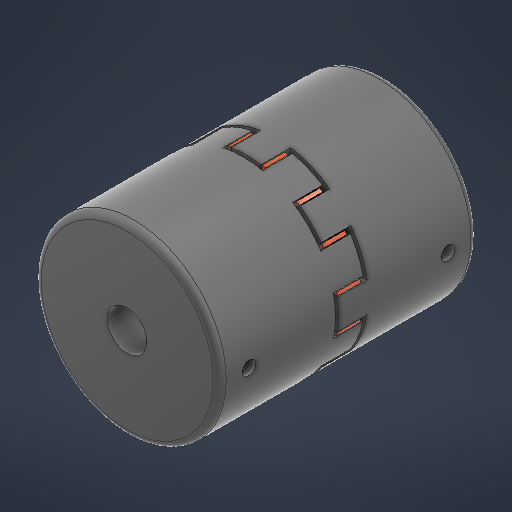
# Autodesk Inventor part: Accouplement12-25
Saved by Autodesk Inventor 2026.2 (Build 302298010, 298A)
## iProperties
Created: 2026-04-18
Part Number: Accouplement12-25
Material: Générique
Document SubType Name: Modeling
Designer: romai
Density: 1 g/cm^3
Appearance: Par défaut
Author: romai
Autodesk Inventor part; units mm, degrees
note: some values were not read from the file. Chosen so that the rebuilt part matches the saved one: direction of "Perçage5".
sketch "Esquisse1" plane through (0, 0, 0) normal (0, 0, 1) x (1, 0, 0)
  circle A0 centre (0, 0) radius 28
  dimension "d0" = 56
  constraints: 1 centre point, 1 coincident
  measures "d0" diameter of A0
extrude "Extrusion1" add sketch "Esquisse1" against normal blind 44
sketch "Esquisse2" plane through (0, 0, 0) normal (0, 0, 1) x (1, 0, 0)
  point P0 (0, 0)
  point P1 (0, 0)
  constraints: 1 coincident
hole "Perçage1" at (0, 0, 0) direction (0, 0, -1) diameter 12 depth 22
sketch "Esquisse4" plane through (0, 0, -44) normal (0, 0, -1) x (-1, 0, 0)
  line L0 (-6, 40) -> (6, 40)
  line L1 (6, 40) -> (6, -40)
  line L2 (6, -40) -> (-6, -40)
  line L3 (-6, -40) -> (-6, 40)
  line L4 (-6, 40) -> (6, -40) construction
  line L5 (6, 40) -> (-6, -40) construction
  line L6 (-32.5269, 24.0416) -> (-24.0416, 32.5269)
  line L7 (24.0416, -32.5269) -> (-32.5269, 24.0416)
  line L8 (-24.0416, 32.5269) -> (32.5269, -24.0416)
  line L9 (32.5269, -24.0416) -> (24.0416, -32.5269)
  line L10 (-40, -6) -> (-40, 6)
  line L11 (40, -6) -> (-40, -6)
  line L12 (-40, 6) -> (40, 6)
  line L13 (40, 6) -> (40, -6)
  line L14 (-24.0416, -32.5269) -> (-32.5269, -24.0416)
  line L15 (32.5269, 24.0416) -> (-24.0416, -32.5269)
  line L16 (-32.5269, -24.0416) -> (24.0416, 32.5269)
  line L17 (24.0416, 32.5269) -> (32.5269, 24.0416)
  line L18 (6, -40) -> (-6, -40)
  line L19 (6, 40) -> (6, -40)
  line L20 (-6, -40) -> (-6, 40)
  line L21 (-6, 40) -> (6, 40)
  line L22 (32.5269, -24.0416) -> (24.0416, -32.5269)
  line L23 (-24.0416, 32.5269) -> (32.5269, -24.0416)
  line L24 (24.0416, -32.5269) -> (-32.5269, 24.0416)
  line L25 (-32.5269, 24.0416) -> (-24.0416, 32.5269)
  line L26 (40, 6) -> (40, -6)
  line L27 (-40, 6) -> (40, 6)
  line L28 (40, -6) -> (-40, -6)
  line L29 (-40, -6) -> (-40, 6)
  line L30 (24.0416, 32.5269) -> (32.5269, 24.0416)
  line L31 (-32.5269, -24.0416) -> (24.0416, 32.5269)
  line L32 (32.5269, 24.0416) -> (-24.0416, -32.5269)
  line L33 (-24.0416, -32.5269) -> (-32.5269, -24.0416)
  point P0 (0, 0)
  point P1 (0, 0)
  point P2 (-6, 14.4853)
  point P3 (-14.4853, 6)
  point P4 (-14.4853, -6)
  point P5 (-6, -14.4853)
  point P6 (6, -14.4853)
  point P7 (14.4853, -6)
  point P8 (14.4853, 6)
  point P9 (6, 14.4853)
  dimension "d17" = 12
  dimension "d18" = 80
  dimension "d21" = 360
  constraints: 68 end point, 2 midpoint, 2 parallel, 1 coincident, 1 horizontal, 1 perpendicular, 65 other
  measures "d17" distance of L1.end L2.end
  measures "d18" distance of L0.end L1.end
extrude "Extrusion2" cut sketch "Esquisse4" against normal blind 9
ref_plane "Plan de construction1" through (0, 0, -36) normal (0, 0, -1) x (-1, 0, 0)
sketch "Esquisse7" plane through (0, 0, -36) normal (0, 0, -1) x (-1, 0, 0)
  arc A0 (15.0964, -23.5817) -> (23.5817, -15.0964) centre (0, 0) ccw projected
  line L0 (14.4853, -6) -> (23.5817, -15.0964) projected
  line L1 (27.3496, -6) -> (14.4853, -6) projected
  arc A1 (27.3496, -6) -> (27.3496, 6) centre (0, 0) ccw projected
  line L2 (14.4853, 6) -> (27.3496, 6) projected
  line L3 (23.5817, 15.0964) -> (14.4853, 6) projected
  arc A2 (23.5817, 15.0964) -> (15.0964, 23.5817) centre (0, 0) ccw projected
  line L4 (6, 14.4853) -> (15.0964, 23.5817) projected
  line L5 (6, 27.3496) -> (6, 14.4853) projected
  arc A3 (6, 27.3496) -> (-6, 27.3496) centre (0, 0) ccw projected
  line L6 (-6, 14.4853) -> (-6, 27.3496) projected
  line L7 (-15.0964, 23.5817) -> (-6, 14.4853) projected
  arc A4 (-15.0964, 23.5817) -> (-23.5817, 15.0964) centre (0, 0) ccw projected
  line L8 (-14.4853, 6) -> (-23.5817, 15.0964) projected
  line L9 (-27.3496, 6) -> (-14.4853, 6) projected
  arc A5 (-27.3496, 6) -> (-27.3496, -6) centre (0, 0) ccw projected
  line L10 (-14.4853, -6) -> (-27.3496, -6) projected
  line L11 (-23.5817, -15.0964) -> (-14.4853, -6) projected
  arc A6 (-23.5817, -15.0964) -> (-15.0964, -23.5817) centre (0, 0) ccw projected
  line L12 (-6, -14.4853) -> (-15.0964, -23.5817) projected
  line L13 (-6, -27.3496) -> (-6, -14.4853) projected
  arc A7 (-6, -27.3496) -> (6, -27.3496) centre (0, 0) ccw projected
  line L14 (6, -14.4853) -> (6, -27.3496) projected
  line L15 (15.0964, -23.5817) -> (6, -14.4853) projected
  line L16 (-13.8817, 5.75) -> (-23.4429, 15.3112)
  line L17 (-14.4853, 6) -> (-23.5817, 15.0964) projected
  line L18 (-13.8817, 5.75) -> (-13.1746, 6.4571)
  line L19 (-13.1746, 6.4571) -> (-22.8708, 16.1533)
  arc A8 (-22.8708, 16.1533) -> (-23.4429, 15.3112) centre (0, 0) ccw
  line L20 (-5.75, 13.8817) -> (-15.3112, 23.4429)
  line L21 (-15.0964, 23.5817) -> (-6, 14.4853) projected
  line L22 (-5.75, 13.8817) -> (-6.4571, 13.1746)
  line L23 (-6.4571, 13.1746) -> (-16.1533, 22.8708)
  arc A9 (-15.3112, 23.4429) -> (-16.1533, 22.8708) centre (0, 0) ccw
  line L24 (-13.8817, -4.75) -> (-27.5942, -4.75)
  line L25 (-13.8817, -5.75) -> (-13.8817, -4.75)
  line L26 (-13.8817, -5.75) -> (-27.4032, -5.75)
  arc A10 (-27.5942, -4.75) -> (-27.4032, -5.75) centre (0, 0) ccw
  line L27 (-13.8817, 5.75) -> (-27.4032, 5.75)
  arc A11 (-27.4032, 5.75) -> (-27.5942, 4.75) centre (0, 0) ccw
  line L28 (-13.8817, 4.75) -> (-27.5942, 4.75)
  line L29 (-13.8817, 5.75) -> (-13.8817, 4.75)
  line L30 (-6.4571, -13.1746) -> (-16.1533, -22.8708)
  line L31 (-5.75, -13.8817) -> (-6.4571, -13.1746)
  line L32 (-5.75, -13.8817) -> (-15.3112, -23.4429)
  arc A12 (-16.1533, -22.8708) -> (-15.3112, -23.4429) centre (0, 0) ccw
  line L33 (-13.8817, -5.75) -> (-23.4429, -15.3112)
  arc A13 (-23.4429, -15.3112) -> (-22.8708, -16.1533) centre (0, 0) ccw
  line L34 (-13.1746, -6.4571) -> (-22.8708, -16.1533)
  line L35 (-13.8817, -5.75) -> (-13.1746, -6.4571)
  line L36 (4.75, -13.8817) -> (4.75, -27.5942)
  line L37 (5.75, -13.8817) -> (4.75, -13.8817)
  line L38 (5.75, -13.8817) -> (5.75, -27.4032)
  arc A14 (4.75, -27.5942) -> (5.75, -27.4032) centre (0, 0) ccw
  line L39 (-5.75, -13.8817) -> (-5.75, -27.4032)
  arc A15 (-5.75, -27.4032) -> (-4.75, -27.5942) centre (0, 0) ccw
  line L40 (-4.75, -13.8817) -> (-4.75, -27.5942)
  line L41 (-5.75, -13.8817) -> (-4.75, -13.8817)
  line L42 (13.1746, -6.4571) -> (22.8708, -16.1533)
  line L43 (13.8817, -5.75) -> (13.1746, -6.4571)
  line L44 (13.8817, -5.75) -> (23.4429, -15.3112)
  arc A16 (22.8708, -16.1533) -> (23.4429, -15.3112) centre (0, 0) ccw
  line L45 (5.75, -13.8817) -> (15.3112, -23.4429)
  arc A17 (15.3112, -23.4429) -> (16.1533, -22.8708) centre (0, 0) ccw
  line L46 (6.4571, -13.1746) -> (16.1533, -22.8708)
  line L47 (5.75, -13.8817) -> (6.4571, -13.1746)
  line L48 (13.8817, 4.75) -> (27.5942, 4.75)
  line L49 (13.8817, 5.75) -> (13.8817, 4.75)
  line L50 (13.8817, 5.75) -> (27.4032, 5.75)
  arc A18 (27.5942, 4.75) -> (27.4032, 5.75) centre (0, 0) ccw
  line L51 (13.8817, -5.75) -> (27.4032, -5.75)
  arc A19 (27.4032, -5.75) -> (27.5942, -4.75) centre (0, 0) ccw
  line L52 (13.8817, -4.75) -> (27.5942, -4.75)
  line L53 (13.8817, -5.75) -> (13.8817, -4.75)
  line L54 (6.4571, 13.1746) -> (16.1533, 22.8708)
  line L55 (5.75, 13.8817) -> (6.4571, 13.1746)
  line L56 (5.75, 13.8817) -> (15.3112, 23.4429)
  arc A20 (16.1533, 22.8708) -> (15.3112, 23.4429) centre (0, 0) ccw
  line L57 (13.8817, 5.75) -> (23.4429, 15.3112)
  arc A21 (23.4429, 15.3112) -> (22.8708, 16.1533) centre (0, 0) ccw
  line L58 (13.1746, 6.4571) -> (22.8708, 16.1533)
  line L59 (13.8817, 5.75) -> (13.1746, 6.4571)
  line L60 (-4.75, 13.8817) -> (-4.75, 27.5942)
  line L61 (-5.75, 13.8817) -> (-4.75, 13.8817)
  line L62 (-5.75, 13.8817) -> (-5.75, 27.4032)
  arc A22 (-4.75, 27.5942) -> (-5.75, 27.4032) centre (0, 0) ccw
  line L63 (5.75, 13.8817) -> (5.75, 27.4032)
  arc A23 (5.75, 27.4032) -> (4.75, 27.5942) centre (0, 0) ccw
  line L64 (4.75, 13.8817) -> (4.75, 27.5942)
  line L65 (5.75, 13.8817) -> (4.75, 13.8817)
  point P0 (-22.8708, -16.1533)
  point P1 (-27.5942, 4.75)
  point P2 (-4.75, -27.5942)
  point P3 (16.1533, -22.8708)
  point P4 (27.5942, -4.75)
  point P5 (22.8708, 16.1533)
  point P6 (4.75, 27.5942)
  dimension "d47" = 1
  dimension "d48" = 0.25
  dimension "d49" = 1
  dimension "d50" = 0.25
  dimension "d69" = 360
  constraints: 96 end point, 36 point on circle, 16 centre point, 9 coincident, 2 parallel, 2 perpendicular, 145 other
  measures "d47" distance of L16.start L18.end
  measures "d48" distance between parallel lines of L8 L16
  measures "d49" distance of L20.start L22.end
  measures "d50" distance between parallel lines of L20 L7
extrude "Extrusion5" add sketch "Esquisse7" along normal blind 7 contours L45 L47 L46 A0 | L38 A7 L36 L37 | L42 L43 L44 A0 | L53 L52 A1 L51 | A7 L39 L41 L40 | L32 A6 L30 L31 | L48 L49 L50 A1 | L59 L58 A2 L57 | A6 L33 L35 L34 | L26 A5 L24 L25 | L54 L55 L56 A2 | L65 L64 A3 L63 | A5 L27 L29 L28 | L16 A4 L19 L18 | L60 L61 L62 A3 | L22 L23 A4 L20
sketch "Esquisse8" plane through (0, 0, -36) normal (0, 0, -1) x (-1, 0, 0)
  arc A0 (15.0964, -23.5817) -> (23.5817, -15.0964) centre (0, 0) ccw projected
  line L0 (14.4853, -6) -> (23.5817, -15.0964) projected
  line L1 (27.3496, -6) -> (14.4853, -6) projected
  arc A1 (27.3496, -6) -> (27.3496, 6) centre (0, 0) ccw projected
  line L2 (14.4853, 6) -> (27.3496, 6) projected
  line L3 (23.5817, 15.0964) -> (14.4853, 6) projected
  arc A2 (23.5817, 15.0964) -> (15.0964, 23.5817) centre (0, 0) ccw projected
  line L4 (6, 14.4853) -> (15.0964, 23.5817) projected
  line L5 (6, 27.3496) -> (6, 14.4853) projected
  arc A3 (6, 27.3496) -> (-6, 27.3496) centre (0, 0) ccw projected
  line L6 (-6, 14.4853) -> (-6, 27.3496) projected
  line L7 (-15.0964, 23.5817) -> (-6, 14.4853) projected
  arc A4 (-15.0964, 23.5817) -> (-23.5817, 15.0964) centre (0, 0) ccw projected
  line L8 (-14.4853, 6) -> (-23.5817, 15.0964) projected
  line L9 (-27.3496, 6) -> (-14.4853, 6) projected
  arc A5 (-27.3496, 6) -> (-27.3496, -6) centre (0, 0) ccw projected
  line L10 (-14.4853, -6) -> (-27.3496, -6) projected
  line L11 (-23.5817, -15.0964) -> (-14.4853, -6) projected
  arc A6 (-23.5817, -15.0964) -> (-15.0964, -23.5817) centre (0, 0) ccw projected
  line L12 (-6, -14.4853) -> (-15.0964, -23.5817) projected
  line L13 (-6, -27.3496) -> (-6, -14.4853) projected
  arc A7 (-6, -27.3496) -> (6, -27.3496) centre (0, 0) ccw projected
  line L14 (6, -14.4853) -> (6, -27.3496) projected
  line L15 (15.0964, -23.5817) -> (6, -14.4853) projected
  line L16 (16.3596, 22.7236) -> (2.535, 8.899)
  line L17 (2.535, 8.899) -> (8.899, 2.535)
  line L18 (8.899, 2.535) -> (22.7236, 16.3596)
  line L19 (6.0129, 12.7304) -> (16.1533, 22.8708) projected
  line L20 (22.8708, 16.1533) -> (9.4636, 2.7461) projected
  arc A8 (22.7236, 16.3596) -> (16.3596, 22.7236) centre (0, 0) ccw
  line L21 (4.5, 8.0851) -> (4.5, 27.636)
  arc A9 (4.5, 27.636) -> (-4.5, 27.636) centre (0, 0) ccw
  line L22 (-4.5, 27.636) -> (-4.5, 8.0851)
  line L23 (-4.5, 8.0851) -> (4.5, 8.0851)
  line L24 (-2.535, 8.899) -> (-16.3596, 22.7236)
  arc A10 (-16.3596, 22.7236) -> (-22.7236, 16.3596) centre (0, 0) ccw
  line L25 (-22.7236, 16.3596) -> (-8.899, 2.535)
  line L26 (-8.899, 2.535) -> (-2.535, 8.899)
  line L27 (-8.0851, 4.5) -> (-27.636, 4.5)
  arc A11 (-27.636, 4.5) -> (-27.636, -4.5) centre (0, 0) ccw
  line L28 (-27.636, -4.5) -> (-8.0851, -4.5)
  line L29 (-8.0851, -4.5) -> (-8.0851, 4.5)
  line L30 (-8.899, -2.535) -> (-22.7236, -16.3596)
  arc A12 (-22.7236, -16.3596) -> (-16.3596, -22.7236) centre (0, 0) ccw
  line L31 (-16.3596, -22.7236) -> (-2.535, -8.899)
  line L32 (-2.535, -8.899) -> (-8.899, -2.535)
  line L33 (-4.5, -8.0851) -> (-4.5, -27.636)
  arc A13 (-4.5, -27.636) -> (4.5, -27.636) centre (0, 0) ccw
  line L34 (4.5, -27.636) -> (4.5, -8.0851)
  line L35 (4.5, -8.0851) -> (-4.5, -8.0851)
  line L36 (2.535, -8.899) -> (16.3596, -22.7236)
  arc A14 (16.3596, -22.7236) -> (22.7236, -16.3596) centre (0, 0) ccw
  line L37 (22.7236, -16.3596) -> (8.899, -2.535)
  line L38 (8.899, -2.535) -> (2.535, -8.899)
  line L39 (8.0851, -4.5) -> (27.636, -4.5)
  arc A15 (27.636, -4.5) -> (27.636, 4.5) centre (0, 0) ccw
  line L40 (27.636, 4.5) -> (8.0851, 4.5)
  line L41 (8.0851, 4.5) -> (8.0851, -4.5)
  point P0 (-4.5, 27.636)
  point P1 (-22.7236, 16.3596)
  point P2 (-27.636, 4.5)
  point P3 (-27.636, -4.5)
  point P4 (-22.7236, -16.3596)
  point P5 (-16.3596, -22.7236)
  point P6 (-4.5, -27.636)
  point P7 (4.5, -27.636)
  point P8 (16.3596, -22.7236)
  point P9 (22.7236, -16.3596)
  point P10 (27.636, -4.5)
  point P11 (27.636, 4.5)
  dimension "d57" = 0.25
  dimension "d58" = 0.25
  dimension "d61" = 360
  constraints: 48 end point, 18 point on circle, 8 centre point, 2 perpendicular, 73 other
  measures "d57" distance between parallel lines of L19 L16
  measures "d58" distance between parallel lines of L20 L18
extrude "Extrusion6" add sketch "Esquisse8" along normal blind 9 contours L36 L34 L35 L38 L41 L39 L37 A0 | L36 L38 L35 L34 | L34 A7 L33 L31 L32 L35 L38 L36 | L39 L41 L38 L37 | L37 L38 L41 L17 L18 L40 A1 L39 | L33 L35 L32 L31 | L31 A6 L30 L28 L29 L32 L35 L33 | L41 L40 L18 L17 | L17 L23 L21 L16 A2 L18 L40 L41 | L32 L30 L28 A5 L27 L25 L26 L29 | L29 L28 L30 L32 | L23 L26 L24 L22 A3 L21 L16 L17 | L17 L16 L21 L23 | L29 L27 L25 A4 L24 L22 L23 L26 | L26 L25 L27 L29 | L23 L22 L24 L26
sketch "Esquisse10" plane through (0, 0, -45) normal (0, 0, -1) x (-1, 0, 0)
  circle A0 centre (0, 0) radius 28
  constraints: 1 centre point, 1 coincident
extrude "Extrusion8" add sketch "Esquisse10" along normal blind 33
sketch "Esquisse11" plane through (0, 0, -78) normal (0, 0, -1) x (-1, 0, 0)
  point P0 (0, 0)
  point P1 (0, 0)
  constraints: 1 coincident
hole "Perçage3" at (0, 0, -78) direction (0, 0, 1) diameter 25 depth 22
ref_plane "Plan de construction2" through (28, 0, -36) normal (1, 0, 0) x (0, 1, 0)
sketch "Esquisse13" plane through (28, 0, -36) normal (1, 0, 0) x (0, 1, 0)
  point P0 (0, 36)
  point P1 (-0.2691, 27.0762)
hole "Perçage5" at (28, -0.2691, -8.9238) direction (-1, 0, 0) diameter 4.134 end up to surface thread size "M5x0.8" class "6H" standard "ISO Metric profile"
ref_plane "Plan de construction3" through (0, 0, -39) normal (0, 0, 1) x (1, 0, 0)
mirror "Mise en miroir1" about plane through (0, 0, -39) normal (0, 0, 1) of "Perçage5"
fillet "Congé1" radius 2 2 edges at (-28, 0, 0) (28, 0, -78)
